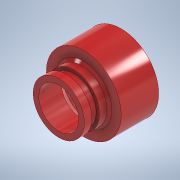
# Autodesk Inventor part: Adaptador_inflador_corrugadoscf
Saved by Autodesk Inventor 2020 (Build 240168000, 168)
## iProperties
Created: 2020-06-10
Part Number: Adaptador_inflador_corrugadoscf
Material: Polyethylene, High Density
Document SubType Name: Modeling
Designer: Juan
Density: 0.952 g/cm^3
Appearance: Red
Author: Juan
Autodesk Inventor part; units mm, degrees
ref_plane "YZ Plane" through (0, 0, 0) normal (1, 0, 0) x (0, 1, 0)
ref_plane "XZ Plane" through (0, 0, 0) normal (0, 1, 0) x (-1, 0, 0)
ref_plane "XY Plane" through (0, 0, 0) normal (0, 0, 1) x (1, 0, 0)
sketch "Sketch1" plane through (0, 0, 0) normal (1, 0, 0) x (0, 1, 0)
  line L0 (0, 0) -> (0, 10) construction
  line L1 (0, 0) -> (0, -15) construction
  line L2 (0, 10) -> (8, 10) construction
  line L3 (0, -15) -> (12.5, -15) construction
  line L4 (8, 10) -> (10.25, 10)
  line L5 (10.25, 10) -> (10.25, 7)
  line L6 (10.25, 7) -> (9, 7)
  line L7 (9, 7) -> (9, 4)
  line L8 (9, 4) -> (10.25, 4)
  line L9 (10.25, 4) -> (10.25, 1)
  line L10 (10.25, 0) -> (15, 0)
  line L11 (12.5, -15) -> (12.5, -12)
  line L12 (12.5, -12) -> (13.5, -12)
  line L13 (8, 10) -> (8, 4)
  line L14 (8, 4) -> (8, 1)
  line L15 (8, 1) -> (12.5, -3.5)
  line L16 (8, 1) -> (14.364, 1) construction
  line L17 (13.5, -12) -> (13.5, -9)
  line L18 (13.5, -9) -> (12.5, -9)
  line L19 (12.5, -9) -> (12.5, -3.5)
  line L20 (15, 0) -> (15, -15)
  line L21 (15, -15) -> (12.5, -15)
  line L22 (10.25, 1) -> (11.25, 0)
  line L23 (10.25, 1) -> (11.6642, 1) construction
  dimension "d1" = 10
  dimension "d2" = 15
  dimension "d3" = 8
  dimension "d4" = 12.5
  dimension "d5" = 2.25
  dimension "d6" = 3
  dimension "d7" = 1.25
  dimension "d8" = 3
  dimension "d9" = 4
  dimension "d10" = 4.75
  dimension "d13" = 3
  dimension "d17" = 6
  dimension "d18" = 3
  dimension "d19" = 45
  dimension "d20" = 3
  dimension "d21" = 15
  dimension "d22" = 45
  constraints: 48 end point, 8 perpendicular, 6 horizontal, 5 point on line, 5 vertical, 2 equal length
  measures "d1" distance of L0.start L0.end
  measures "d2" distance of L0.start L1.end
  measures "d3" distance of L0.end L2.end
  measures "d4" distance of L1.end L3.end
  measures "d5" distance of L2.end L4.end
  measures "d6" distance of L4.end L5.end
  measures "d7" distance of L5.end L6.end
  measures "d8" distance of L6.end L7.end
  measures "d9" distance of L8.end L10.start
  measures "d10" distance of L10.start L10.end
  measures "d13" distance of L3.end L11.end
  measures "d17" distance of L2.end L13.end
  measures "d18" distance of L13.end L14.end
  measures "d19" angle of L15 L16
  measures "d20" distance of L12.end L17.end
  measures "d21" distance of L10.end L20.end
  measures "d22" angle of L22 L23
revolve "Revolution1" add sketch "Sketch1" angle 360 about axis through (0, 0, 0) along (0, 0, -1)
body "Solid1"
